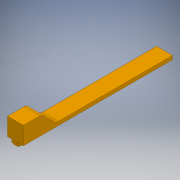
# Autodesk Inventor part: 20X20Connector
Saved by Autodesk Inventor 2017 (Build 210142000, 142)
## iProperties
Created: 2018-01-13
Part Number: 20X20Connector
Material: Generic
Document SubType Name: Modeling
Designer: User
Density: 1 g/cm^3
Appearance: Default(1)
Author: User
Autodesk Inventor part; units mm, degrees
ref_plane "YZ Plane" through (0, 0, 0) normal (1, 0, 0) x (0, 1, 0)
ref_plane "XZ Plane" through (0, 0, 0) normal (0, 1, 0) x (-1, 0, 0)
ref_plane "XY Plane" through (0, 0, 0) normal (0, 0, 1) x (1, 0, 0)
sketch "Sketch1" plane through (0, 0, 0) normal (0, 0, 1) x (1, 0, 0)
  line L0 (-8.7854, 4.1412) -> (7.7246, 4.1412)
  line L1 (7.7246, 1.6412) -> (1.8496, 1.6412)
  line L2 (1.8496, 1.6412) -> (1.8496, -0.3588)
  line L3 (1.8496, -0.3588) -> (5.4596, -0.3588)
  line L4 (2.5721, -3.1588) -> (-3.1429, -3.1588)
  line L5 (-3.1429, -3.1588) -> (-6.0304, -1.1208)
  line L6 (-6.0304, -1.1208) -> (-6.0304, -0.3588)
  line L7 (-6.0304, -0.3588) -> (-2.9104, -0.3588)
  line L8 (-2.9104, -0.3588) -> (-2.9104, 1.6412)
  line L9 (-2.9104, 1.6412) -> (-8.7854, 1.6412)
  line L10 (-8.7854, 1.6412) -> (-8.7854, 4.1412)
  line L11 (5.4596, -0.3588) -> (5.4596, -1.1208)
  line L12 (5.4596, -1.1208) -> (2.5721, -3.1588)
  line L13 (7.7246, 4.1412) -> (7.7246, 1.6412)
  point P0 (0, 0)
  dimension "d0" = 2.5
  dimension "d1" = 2
  dimension "d2" = 4.76
  dimension "d3" = 11.49
  dimension "d4" = 2.755
  dimension "d5" = 5.715
  dimension "d6" = 5.6425
  dimension "d7" = 5.875
  dimension "d8" = 0.762
  dimension "d9" = 0.762
  dimension "d11" = 144.786
  dimension "d12" = 2.8875
  dimension "d14" = 16.51
  constraints: 28 end point, 5 perpendicular, 4 point on line, 1 horizontal, 1 vertical
  measures "d0" distance between parallel lines of L9 L0
  measures "d1" distance between parallel lines of L7 L9
  measures "d2" distance between parallel lines of L2 L8
  measures "d3" distance between parallel lines of L6 L11
  measures "d4" distance between parallel lines of L6 L10
  measures "d5" distance of L4.start L4.end
  measures "d6" distance from line of L4.end L10
  measures "d7" distance between parallel lines of L10 L8
  measures "d8" distance of L5.end L6.end
  measures "d9" distance of L3.end L11.end
  measures "d11" angle of L12 L4
  measures "d12" distance from line of L4.start L11
  measures "d14" distance between parallel lines of L13 L10
extrude "Extrusion1" add sketch "Sketch1" along normal blind 25.4
ref_plane "Work Plane1" through (-8.7854, 4.1412, 0) normal (0, 1, 0) x (1, 0, 0)
fillet "Fillet2" radius 0.3969 4 edges at (1.8496, -0.3588, 12.7) (1.8496, 1.6412, 12.7) (-2.9104, 1.6412, 12.7) (-2.9104, -0.3588, 12.7)
sketch "Sketch2" plane through (0, 0, 25.4) normal (0, 0, 1) x (1, 0, 0)
  line L0 (-8.7854, 4.1412) -> (7.7246, 4.1412) projected
  line L1 (-8.7854, 4.1412) -> (7.7246, 4.1412)
  line L2 (2.2465, 1.6412) -> (7.7246, 1.6412) projected
  line L3 (7.7246, 4.1412) -> (7.7246, 1.6412)
  line L4 (7.7246, 1.6412) -> (1.8496, 1.6412)
  line L5 (1.8496, 1.6412) -> (1.8496, -0.3588)
  line L6 (5.4596, -0.3588) -> (2.2465, -0.3588) projected
  line L7 (1.8496, -0.3588) -> (5.4596, -0.3588)
  line L8 (5.4596, -1.1208) -> (5.4596, -0.3588) projected
  line L9 (5.4596, -0.3588) -> (5.4596, -1.1208)
  line L10 (5.4596, -1.1208) -> (2.6967, -3.1588)
  line L11 (-3.1429, -3.1588) -> (2.5721, -3.1588) projected
  line L12 (2.5721, -3.1588) -> (5.4596, -1.1208)
  line L13 (-3.1429, -3.1588) -> (2.5721, -3.1588)
  line L14 (-8.7854, 4.1412) -> (-8.7854, 1.6412) projected
  line L15 (-8.7854, 4.1412) -> (-8.7854, 1.6412)
  line L16 (-8.7854, 1.6412) -> (-2.9339, 1.6412)
  line L17 (-2.9339, 1.6412) -> (-2.9339, -0.3584)
  line L18 (-2.9339, -0.3584) -> (-6.0304, -0.3584)
  line L19 (-6.0304, -1.1208) -> (-3.1429, -3.1588) projected
  line L20 (-6.0304, -0.3584) -> (-6.0304, -1.1208)
  line L21 (-6.0304, -1.1208) -> (-3.1429, -3.1588)
  point P0 (0, 0)
  constraints: 30 end point, 9 perpendicular, 2 collinear, 2 point on line, 1 vertical
extrude "Extrusion2" add sketch "Sketch2" along normal blind 177.8
sketch "Sketch3" plane through (-8.7854, 1.6412, 0) normal (-1, 0, 0) x (0, 0, 1)
  line L0 (0, 0) -> (0, 2.5) projected
  line L1 (0, 0) -> (0, 2.5)
  point P0 (0, -1.6412)
  constraints: 2 end point, 1 collinear
sketch "Sketch4" plane through (-8.7854, 4.1412, 0) normal (0, 1, 0) x (1, 0, 0)
  line L0 (0, 0) -> (16.51, 0) projected
  line L1 (0, 0) -> (0, -203.2) projected
  line L2 (16.51, 0) -> (0, 0)
  line L3 (0, 0) -> (0, -203.2)
  line L4 (0, -203.2) -> (16.51, -203.2)
  line L5 (16.51, -203.2) -> (16.51, 0)
  point P0 (8.7854, 0)
  constraints: 8 end point, 2 parallel, 1 horizontal, 1 perpendicular
extrude "Extrusion3" add sketch "Sketch4" along normal blind 2.54
fillet "Fillet3" radius 0.3962 4 edges at (1.8496, 1.6412, 114.3) (1.8496, -0.3588, 114.3) (-2.9339, 1.6412, 114.3) (-2.9339, -0.3584, 114.3)
sketch "Sketch5" plane through (-8.7854, 6.6812, 0) normal (0, 1, 0) x (1, 0, 0)
  line L0 (0, -203.2) -> (16.51, -203.2) projected
  line L1 (0, 0) -> (0, -203.2) projected
  line L2 (16.51, -203.2) -> (0, -203.2)
  line L3 (0, -203.2) -> (0, -177.8)
  line L4 (0, -177.8) -> (16.51, -177.8)
  line L5 (16.51, -177.8) -> (16.51, -203.2)
  point P0 (8.7854, 0)
  dimension "d25" = 25.4
  constraints: 8 end point, 2 parallel, 1 horizontal, 1 perpendicular, 1 point on line
  measures "d25" distance of L2.end L3.end
extrude "Extrusion4" add sketch "Sketch5" along normal blind 19.05
chamfer "Chamfer1" distance 19.05 angle 45 1 edges at (-0.5304, 6.6812, 177.8)
sketch "Sketch6" plane through (7.7246, 1.6412, 203.2) normal (1, 0, 0) x (0, 0, -1)
  line L0 (0, 0) -> (0, 24.09) projected
  line L1 (0, 24.09) -> (0, 0)
  line L2 (203.2, 5.04) -> (203.2, 0) projected
  line L3 (0, 0) -> (203.2, 0)
  line L4 (203.2, 0) -> (203.2, 5.04)
  line L5 (44.45, 5.04) -> (203.2, 5.04) projected
  line L6 (203.2, 5.04) -> (44.45, 5.04)
  line L7 (0, 24.09) -> (25.4, 24.09) projected
  line L8 (44.45, 5.04) -> (25.4, 24.09)
  line L9 (25.4, 24.09) -> (0, 24.09)
  point P0 (203.2, -1.6412)
  constraints: 12 end point, 4 collinear, 1 perpendicular
extrude "Extrusion5" add sketch "Sketch6" along normal blind 2.54
sketch "Sketch7" plane through (-8.7854, 1.6412, 0) normal (-1, 0, 0) x (0, 0, 1)
  line L0 (203.2, 0) -> (0, 0) projected
  line L1 (0, 0) -> (0, 5.04) projected
  line L2 (0, 0) -> (0, 5.04)
  line L3 (158.75, 5.04) -> (177.8, 24.09) projected
  line L4 (0, 5.04) -> (158.75, 5.04)
  line L5 (177.8, 24.09) -> (203.2, 24.09) projected
  line L6 (158.75, 5.04) -> (177.8, 24.09)
  line L7 (177.8, 24.09) -> (203.2, 24.09)
  line L8 (25.4, 0) -> (203.2, 0) projected
  line L9 (203.2, 24.09) -> (203.2, 0)
  line L10 (203.2, 0) -> (0, 0)
  point P0 (0, -1.6412)
  constraints: 12 end point, 2 collinear, 2 perpendicular, 1 vertical
extrude "Extrusion6" add sketch "Sketch7" along normal blind 2.54
fillet "Fillet4" radius 6.35 7 edges at (-10.0554, 25.7312, 177.8) (-0.5304, 25.7312, 177.8) (8.9946, 25.7312, 177.8) (-0.5304, 25.7311, 177.8) (-10.0554, 6.6812, 158.75) (8.9946, 6.6812, 158.75) (-0.5304, 6.6812, 158.7501)
equation "\"d4\" = -0.5 * d3 + 0.5 * d13"
equation "\"d6\" = -0.5 * d5 + 0.5 * d13"
equation "\"d7\" = -0.5 * d2 + 0.5 * d14"
equation "\"d9\" = d8"
equation "\"d13\" = 17"
body "Solid1"
